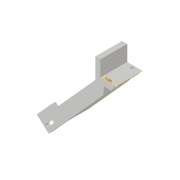
# Autodesk Inventor part: arm stop
Saved by Autodesk Inventor 2018 (Build 220112000, 112)
## iProperties
Created: 2018-12-28
Part Number: arm stop
Material: Generic
Document SubType Name: Modeling
Designer: ball
Density: 1 g/cm^3
Appearance: Default
Author: ball
Autodesk Inventor part; units mm, degrees
ref_plane "YZ Plane" through (0, 0, 0) normal (1, 0, 0) x (0, 1, 0)
ref_plane "XZ Plane" through (0, 0, 0) normal (0, 1, 0) x (-1, 0, 0)
ref_plane "Work Plane1" through (0, 0, 0) normal (0, 0, 1) x (1, 0, 0)
sketch "Sketch1" plane through (0, 0, 0) normal (0, 0, 1) x (1, 0, 0)
  line L0 (4.129202, -9.5377) -> (6.406797, -9.5377) construction
  line L1 (9.525, -8.41296) -> (9.525, -7.435497) construction
  line L2 (-6.406797, 9.5123) -> (-4.129202, 9.5123) construction
  line L3 (-9.525, 4.116502) -> (-9.525, 6.394097) construction
  line L4 (9.314549, -9.373063) -> (-73.965447, -101.864868) construction
  line L5 (9.166309, -9.5377) -> (-73.965447, -101.864868)
  line L6 (-73.965447, -101.864868) -> (-85.121243, -91.820144)
  line L7 (6.33881, 9.756536) -> (-85.121243, -91.820144) construction
  line L8 (9.166309, -9.5377) -> (-9.997679, -9.5377)
  line L9 (-9.997679, -9.5377) -> (-9.997679, 9.756536)
  line L10 (-9.997679, 9.756536) -> (-16.347679, 9.756536)
  line L11 (-16.347679, 9.756536) -> (-16.347679, -15.439362)
  line L12 (-16.347679, -15.439362) -> (-85.121243, -91.820144)
  point P0 (0, 0)
  dimension "d0" = 124.46
  dimension "d1" = 48
  dimension "d5" = 6.35
  constraints: 26 end point, 4 point on line, 3 horizontal, 3 perpendicular, 2 collinear, 2 vertical, 1 parallel, 8 other
  measures "d0" distance of L4.start L4.end
  measures "d1" angle of L0 L4
  measures "d5" distance of L9.end L10.end
ref_plane "Work Plane2" through (-4.445, -9.144, -33.02) normal (0, 0, -1) x (0, 1, 0)
extrude "Extrusion1" add sketch "Sketch1" against normal up to surface (33.02 mm away)
sketch "Sketch2" plane through (-73.965447, -101.864868, -33.02) normal (-0.6691306, -0.7431448, 0) x (0.7431448, -0.6691306, 0)
  line L0 (0, 33.02) -> (0, 0)
  line L1 (-15.011605, 33.02) -> (-15.011605, 0)
  line L2 (0, 0) -> (-15.011605, 0)
  line L3 (-15.011605, 0) -> (-15.011605, 26.67)
  line L4 (-15.011605, 26.67) -> (0, 26.67)
  line L5 (0, 26.67) -> (0, 0)
  line L6 (-15.011605, 33.02) -> (0, 33.02)
  point P0 (-13.193862, 33.02)
  dimension "d19" = 6.35
  constraints: 8 end point, 2 parallel, 1 horizontal, 1 perpendicular, 1 point on line
  measures "d19" distance between parallel lines of L6 L4
extrude "Extrusion2" cut sketch "Sketch2" against normal blind 25.4 contours L0 L2 L1 L4
sketch "Sketch3" plane through (-73.965447, -101.864868, -6.35) normal (0, 0, -1) x (-0.7431448, 0.6691306, 0)
  line L0 (19.8882, 12.0904) -> (19.8882, 3.175) construction
  line L1 (0, 25.4) -> (15.011605, 25.4) construction
  line L2 (15.011605, 0) -> (0, 0) construction
  line L3 (0, 0) -> (19.8882, 0) construction
  line L4 (19.8882, 0) -> (19.8882, 25.4) construction
  line L5 (19.8882, 25.4) -> (0, 25.4) construction
  line L6 (0, 25.4) -> (0, 0) construction
  line L7 (15.011605, 0) -> (19.8882, 0)
  line L8 (19.8882, 0) -> (19.8882, 25.4)
  line L9 (19.8882, 25.4) -> (15.011605, 25.4)
  line L10 (15.011605, 25.4) -> (15.011605, 0)
  point P0 (13.193862, 125.192894)
  constraints: 18 end point, 4 parallel, 2 horizontal, 2 perpendicular, 1 vertical, 2 other
extrude "Extrusion3" add sketch "Sketch3" against normal up to surface (6.35 mm away)
sketch "Sketch4" plane through (0, 0, 0) normal (0, 0, 1) x (1, 0, 0)
  circle A0 centre (-72.965209, -90.773771) radius 1.1938 construction
  circle A1 centre (-65.459407, -96.637946) radius 1.1938 construction
  line L0 (-72.965209, -90.773771) -> (-64.699827, -81.594134) construction
  line L1 (-88.74526, -88.557064) -> (-71.749342, -69.681186) construction
  line L2 (-72.965209, -90.773771) -> (-77.668593, -95.997407) construction
  line L3 (-76.364393, -94.548947) -> (-69.566026, -86.998595) construction
  line L4 (-75.194088, -95.602693) -> (-68.395721, -88.052342)
  line L5 (-70.73633, -85.944848) -> (-77.534697, -93.4952)
  arc A2 (-77.534697, -93.4952) -> (-75.194088, -95.602693) centre (-76.364393, -94.548947) ccw
  arc A3 (-68.395721, -88.052342) -> (-70.73633, -85.944848) centre (-69.566026, -86.998595) ccw
  line L6 (-65.459407, -96.637946) -> (-57.773123, -88.101463) construction
  line L7 (-73.965447, -101.864868) -> (9.166309, -9.5377) construction
  line L8 (-65.459407, -96.637946) -> (-69.368096, -100.978985) construction
  line L9 (-68.85859, -100.413122) -> (-62.060223, -92.862771) construction
  line L10 (-67.688286, -101.466869) -> (-60.889919, -93.916518)
  line L11 (-63.230528, -91.809024) -> (-70.028895, -99.359375)
  arc A4 (-70.028895, -99.359375) -> (-67.688286, -101.466869) centre (-68.85859, -100.413122) ccw
  arc A5 (-60.889919, -93.916518) -> (-63.230528, -91.809024) centre (-62.060223, -92.862771) ccw
  point P0 (0, 0)
  dimension "d13" = 5.08
  dimension "d14" = 3.1496
  dimension "d15" = 5.08
  dimension "d16" = 3.1496
  constraints: 24 end point, 8 point on circle, 8 tangent, 6 centre point, 6 parallel, 2 midpoint, 2 point on line, 4 other
  measures "d13" distance of L0.start L3.end
  measures "d14" diameter of A3
  measures "d15" distance of L6.start L9.end
  measures "d16" diameter of A5
extrude "Extrusion4" cut sketch "Sketch4" against normal through all
sketch "Sketch5" plane through (-73.965447, -101.864868, -6.35) normal (0, 0, -1) x (-0.7431448, 0.6691306, 0)
  arc A0 (6.7564, 14.73835) -> (3.6068, 14.73835) centre (5.1816, 14.73835) ccw
  arc A1 (3.6068, 4.57835) -> (6.7564, 4.57835) centre (5.1816, 4.57835) ccw
  line L0 (5.1816, 14.73835) -> (5.1816, 4.57835) construction
  line L1 (1.6256, 14.73835) -> (1.6256, 4.57835)
  line L2 (8.7376, 4.57835) -> (8.7376, 14.73835)
  arc A2 (8.7376, 14.73835) -> (1.6256, 14.73835) centre (5.1816, 14.73835) ccw
  arc A3 (1.6256, 4.57835) -> (8.7376, 4.57835) centre (5.1816, 4.57835) ccw
  arc A4 (8.252871, 13.991581) -> (5.103271, 13.991581) centre (6.678071, 13.991581) ccw
  arc A5 (5.103271, 3.831581) -> (8.252871, 3.831581) centre (6.678071, 3.831581) ccw
  line L3 (6.678071, 13.991581) -> (6.678071, 3.831581) construction
  line L4 (3.122071, 13.991581) -> (3.122071, 3.831581)
  line L5 (10.234071, 3.831581) -> (10.234071, 13.991581)
  arc A6 (10.234071, 13.991581) -> (3.122071, 13.991581) centre (6.678071, 13.991581) ccw
  arc A7 (3.122071, 3.831581) -> (10.234071, 3.831581) centre (6.678071, 3.831581) ccw
  point P0 (13.193862, 125.192894)
  point P1 (5.1816, 9.65835)
  point P2 (6.678071, 8.911581)
  dimension "d20" = 7.112
  dimension "d21" = 7.112
  constraints: 16 end point, 8 point on circle, 8 tangent, 4 centre point, 3 parallel, 2 midpoint, 1 vertical
  measures "d20" diameter of A3
  measures "d21" diameter of A7
sketch "Sketch5 outline for Extrusion5" plane through (-73.965447, -101.864868, -6.35) normal (0, 0, -1) x (-0.7431448, 0.6691306, 0)
  line L0 (10.234071, 3.831581) -> (10.234071, 13.991581)
  arc A0 (10.234071, 13.991581) -> (7.473106, 17.457566) centre (6.678071, 13.991581) ccw
  arc A1 (7.473106, 17.457566) -> (1.6256, 14.73835) centre (5.1816, 14.73835) ccw
  line L1 (1.6256, 14.73835) -> (1.6256, 4.57835)
  arc A2 (1.6256, 4.57835) -> (4.386565, 1.112364) centre (5.1816, 4.57835) ccw
  arc A3 (4.386565, 1.112364) -> (10.234071, 3.831581) centre (6.678071, 3.831581) ccw
extrude "Extrusion5" cut sketch "Sketch5 outline for Extrusion5" against normal blind 3.556
sketch "Sketch6" plane through (-9.997679, -9.5377, 0) normal (0, 1, 0) x (1, 0, 0)
  arc A0 (9.506526, 4.79213) -> (10.740649, 4.300966) centre (9.523849, 3.039616) ccw construction
  arc A1 (9.506526, 31.732899) -> (10.740649, 31.241734) centre (9.523849, 29.980384) ccw construction
  circle A2 centre (9.523849, 29.980384) radius 1.9685
  circle A3 centre (9.523849, 3.039616) radius 1.9685
  point P0 (9.997679, 0)
  dimension "d24" = 3.937
  dimension "d25" = 3.937
  constraints: 4 centre point, 4 point on circle, 2 coincident, 8 other
  measures "d24" diameter of A2
  measures "d25" diameter of A3
extrude "Extrusion6" cut sketch "Sketch6" against normal through all
sketch "Sketch7" plane through (9.166309, -9.5377, 0) normal (0.7431448, -0.6691306, 0) x (0, 0, -1)
  line L0 (33.02, -98.838459) -> (33.02, 0) construction
  line L1 (33.02, -9.525) -> (0, -9.525) construction
  point P0 (0, 0.954435)
  constraints: 2 end point, 1 perpendicular, 1 point on line
sketch "Sketch8" plane through (9.166309, -9.5377, -33.02) normal (0, 0, -1) x (-1, 0, 0)
  line L0 (11.608639, 0) -> (11.608639, -12.892699) construction
  line L1 (66.135838, -73.451289) -> (0, 0) construction
  line L2 (11.608639, -7.62) -> (6.861079, -7.62) construction
  line L3 (0, 0) -> (19.163987, 0) construction
  line L4 (7.671639, 0) -> (7.671639, -8.520218) construction
  line L5 (14.910639, 0) -> (14.910639, -14.251905) construction
  line L6 (6.861079, -7.62) -> (14.910639, -7.62)
  line L7 (83.131755, -92.327168) -> (0, 0)
  line L8 (15.69062, -17.426199) -> (6.861079, -7.62)
  line L9 (15.69062, -17.426199) -> (14.910639, -7.62)
  point P0 (9.166309, 9.5377)
  dimension "d28" = 7.62
  dimension "d29" = 3.302
  constraints: 10 end point, 5 point on line, 1 collinear, 1 horizontal, 1 parallel
  measures "d28" distance between parallel lines of L3 L2
  measures "d29" distance between parallel lines of L0 L5
extrude "Extrusion7" cut sketch "Sketch8" against normal blind 8.763
sketch "Sketch9" plane through (0, 0, 0) normal (0, 0, 1) x (1, 0, 0)
  line L0 (2.30523, -17.1577) -> (-5.74433, -17.1577) construction
  line L1 (-5.74433, -17.1577) -> (-6.524312, -26.963899) construction
  line L2 (2.30523, -17.1577) -> (-6.524312, -26.963899)
  line L3 (-73.965447, -101.864868) -> (9.166309, -9.5377)
  line L4 (2.30523, -17.1577) -> (-5.74433, -17.1577)
  line L5 (-5.2705, -26.963899) -> (-5.2705, -17.1577)
  point P0 (0, 0)
  constraints: 4 end point, 1 collinear, 1 vertical
sketch "Sketch9 outline for Extrusion8" plane through (0, 0, 0) normal (0, 0, 1) x (1, 0, 0)
  line L0 (-6.524312, -26.963899) -> (2.30523, -17.1577)
  line L1 (-5.74433, -17.1577) -> (-6.524312, -26.963899)
  line L2 (2.30523, -17.1577) -> (-5.74433, -17.1577)
extrude "Extrusion8" cut sketch "Sketch9 outline for Extrusion8" against normal blind 8.763
body "Solid1"
